Autodesk Fusion 360 part; units mm, degrees
(part 16 of 18)
  line L9589 (199.0354, -77.1606) -> (199.0354, -76.5606)
  line L9590 (199.3854, -77.1606) -> (199.0354, -77.1606)
  line L9591 (199.0354, -76.5606) -> (199.3854, -76.5606)
  line L9592 (195.5854, -58.0978) -> (195.9354, -58.0978)
  line L9593 (195.9354, -58.0978) -> (195.9354, -57.4978)
  line L9594 (195.9354, -57.4978) -> (195.5854, -57.4978)
  line L9595 (195.5854, -57.4978) -> (195.5854, -58.0978)
  line L9596 (199.0354, -57.4978) -> (199.3854, -57.4978)
  line L9597 (199.3854, -58.0978) -> (199.0354, -58.0978)
  line L9598 (199.3854, -57.4978) -> (199.3854, -58.0978)
  line L9599 (199.0354, -58.0978) -> (199.0354, -57.4978)
  line L9600 (195.5854, -19.385) -> (195.5854, -19.985)
  line L9601 (195.9354, -19.385) -> (195.5854, -19.385)
  line L9602 (195.9354, -19.985) -> (195.9354, -19.385)
  line L9603 (195.5854, -19.985) -> (195.9354, -19.985)
  line L9604 (199.3854, -19.985) -> (199.0354, -19.985)
  line L9605 (199.0354, -19.985) -> (199.0354, -19.385)
  line L9606 (199.3854, -19.385) -> (199.3854, -19.985)
  line L9607 (199.0354, -19.385) -> (199.3854, -19.385)
  line L9608 (203.2384, -3.41) -> (203.2384, -4.21)
  line L9609 (202.9384, -3.41) -> (203.2384, -3.41)
  line L9610 (202.9384, -4.21) -> (202.9384, -3.41)
  line L9611 (203.2384, -4.21) -> (202.9384, -4.21)
  line L9612 (201.9384, -4.21) -> (201.9384, -3.41)
  line L9613 (201.6384, -4.21) -> (201.9384, -4.21)
  line L9614 (201.6384, -3.41) -> (201.6384, -4.21)
  line L9615 (201.9384, -3.41) -> (201.6384, -3.41)
  line L9616 (201.0334, -7.131) -> (201.0334, -6.331)
  line L9617 (201.0334, -6.331) -> (201.3334, -6.331)
  line L9618 (201.3334, -6.331) -> (201.3334, -7.131)
  line L9619 (201.3334, -7.131) -> (201.0334, -7.131)
  line L9620 (199.7334, -7.131) -> (200.0334, -7.131)
  line L9621 (199.7334, -6.331) -> (199.7334, -7.131)
  line L9622 (200.0334, -7.131) -> (200.0334, -6.331)
  line L9623 (200.0334, -6.331) -> (199.7334, -6.331)
  line L9624 (204.9404, -4.426) -> (205.2404, -4.426)
  line L9625 (204.9404, -5.226) -> (204.9404, -4.426)
  line L9626 (205.2404, -4.426) -> (205.2404, -5.226)
  line L9627 (205.2404, -5.226) -> (204.9404, -5.226)
  line L9628 (206.5404, -5.226) -> (206.5404, -4.426)
  line L9629 (206.2404, -4.426) -> (206.2404, -5.226)
  line L9630 (206.5404, -4.426) -> (206.2404, -4.426)
  line L9631 (206.2404, -5.226) -> (206.5404, -5.226)
  line L9632 (2.9129, -0.5611) -> (1.413, -0.5611)
  line L9633 (2.9129, 0.6389) -> (2.9129, -0.5611)
  line L9634 (1.413, 0.6389) -> (2.9129, 0.6389)
  line L9635 (1.413, -0.5611) -> (1.413, 0.6389)
  line L9636 (2.9129, -10.3611) -> (2.9129, -11.5611)
  line L9637 (1.413, -11.5611) -> (1.413, -10.3611)
  line L9638 (1.413, -10.3611) -> (2.9129, -10.3611)
  line L9639 (2.9129, -11.5611) -> (1.413, -11.5611)
  line L9640 (197.1222, -3.92) -> (197.1222, -3.67)
  line L9641 (197.4822, -3.92) -> (197.1222, -3.92)
  line L9642 (197.1222, -3.67) -> (197.4822, -3.67)
  line L9643 (197.4822, -3.67) -> (197.4822, -3.92)
  line L9644 (197.4823, -4.97) -> (197.4823, -5.22)
  line L9645 (197.4823, -5.22) -> (197.1223, -5.22)
  line L9646 (197.1223, -5.22) -> (197.1223, -4.97)
  line L9647 (197.1223, -4.97) -> (197.4823, -4.97)
  line L9648 (195.5524, -3.92) -> (195.1924, -3.92)
  line L9649 (195.5524, -3.67) -> (195.5524, -3.92)
  line L9650 (195.1924, -3.67) -> (195.5524, -3.67)
  line L9651 (195.1924, -3.92) -> (195.1924, -3.67)
  line L9652 (195.1924, -4.57) -> (195.1924, -4.32)
  line L9653 (195.5524, -4.32) -> (195.5524, -4.57)
  line L9654 (195.1924, -4.32) -> (195.5524, -4.32)
  line L9655 (195.5524, -4.57) -> (195.1924, -4.57)
  line L9656 (195.5524, -4.97) -> (195.5524, -5.22)
  line L9657 (195.5524, -5.22) -> (195.1924, -5.22)
  line L9658 (195.1924, -4.97) -> (195.5524, -4.97)
  line L9659 (195.1924, -5.22) -> (195.1924, -4.97)
  line L9660 (201.1604, -2.305) -> (201.1604, -1.505)
  line L9661 (201.1604, -1.505) -> (201.4604, -1.505)
  line L9662 (201.4604, -1.505) -> (201.4604, -2.305)
  line L9663 (201.4604, -2.305) -> (201.1604, -2.305)
  line L9664 (199.8604, -2.305) -> (200.1604, -2.305)
  line L9665 (200.1604, -1.505) -> (199.8604, -1.505)
  line L9666 (200.1604, -2.305) -> (200.1604, -1.505)
  line L9667 (199.8604, -1.505) -> (199.8604, -2.305)
  line L9668 (207.5745, -6.0629) -> (207.9745, -6.0629)
  line L9669 (207.9745, -6.2629) -> (207.5745, -6.2629)
  line L9670 (207.9745, -6.0629) -> (207.9745, -6.2629)
  line L9671 (207.5745, -6.2629) -> (207.5745, -6.0629)
  line L9672 (207.9745, -6.6629) -> (207.5745, -6.6629)
  line L9673 (207.5745, -6.6629) -> (207.5745, -6.4629)
  line L9674 (207.5745, -6.4629) -> (207.9745, -6.4629)
  line L9675 (207.9745, -6.4629) -> (207.9745, -6.6629)
  line L9676 (207.5745, -6.8629) -> (207.9745, -6.8629)
  line L9677 (207.9745, -6.8629) -> (207.9745, -7.0629)
  line L9678 (207.5745, -7.0629) -> (207.5745, -6.8629)
  line L9679 (207.9745, -7.0629) -> (207.5745, -7.0629)
  line L9680 (207.5745, -7.2629) -> (207.9745, -7.2629)
  line L9681 (207.9745, -7.2629) -> (207.9745, -7.4629)
  line L9682 (207.5745, -7.4629) -> (207.5745, -7.2629)
  line L9683 (207.9745, -7.4629) -> (207.5745, -7.4629)
  line L9684 (207.5745, -7.8629) -> (207.5745, -7.6629)
  line L9685 (207.9745, -7.8629) -> (207.5745, -7.8629)
  line L9686 (207.9745, -7.6629) -> (207.9745, -7.8629)
  line L9687 (207.5745, -7.6629) -> (207.9745, -7.6629)
  line L9688 (207.9745, -8.0629) -> (207.9745, -8.2629)
  line L9689 (207.9745, -8.2629) -> (207.5745, -8.2629)
  line L9690 (207.5745, -8.2629) -> (207.5745, -8.0629)
  line L9691 (207.5745, -8.0629) -> (207.9745, -8.0629)
  line L9692 (207.9745, -8.6629) -> (207.5745, -8.6629)
  line L9693 (207.5745, -8.4629) -> (207.9745, -8.4629)
  line L9694 (207.5745, -8.6629) -> (207.5745, -8.4629)
  line L9695 (207.9745, -8.4629) -> (207.9745, -8.6629)
  line L9696 (207.5745, -8.8629) -> (207.9745, -8.8629)
  line L9697 (207.9745, -9.0629) -> (207.5745, -9.0629)
  line L9698 (207.5745, -9.0629) -> (207.5745, -8.8629)
  line L9699 (207.9745, -8.8629) -> (207.9745, -9.0629)
  line L9700 (207.5745, -9.4629) -> (207.5745, -9.2629)
  line L9701 (207.9745, -9.2629) -> (207.9745, -9.4629)
  line L9702 (207.5745, -9.2629) -> (207.9745, -9.2629)
  line L9703 (207.9745, -9.4629) -> (207.5745, -9.4629)
  line L9704 (207.5745, -9.6629) -> (207.9745, -9.6629)
  line L9705 (207.9745, -9.8629) -> (207.5745, -9.8629)
  line L9706 (207.5745, -9.8629) -> (207.5745, -9.6629)
  line L9707 (207.9745, -9.6629) -> (207.9745, -9.8629)
  line L9708 (207.5745, -10.2629) -> (207.5745, -10.0629)
  line L9709 (207.9745, -10.0629) -> (207.9745, -10.2629)
  line L9710 (207.9745, -10.2629) -> (207.5745, -10.2629)
  line L9711 (207.5745, -10.0629) -> (207.9745, -10.0629)
  line L9712 (207.9745, -10.6629) -> (207.5745, -10.6629)
  line L9713 (207.9745, -10.4629) -> (207.9745, -10.6629)
  line L9714 (207.5745, -10.6629) -> (207.5745, -10.4629)
  line L9715 (207.5745, -10.4629) -> (207.9745, -10.4629)
  line L9716 (207.5745, -10.8629) -> (207.9745, -10.8629)
  line L9717 (207.9745, -10.8629) -> (207.9745, -11.0629)
  line L9718 (207.9745, -11.0629) -> (207.5745, -11.0629)
  line L9719 (207.5745, -11.0629) -> (207.5745, -10.8629)
  line L9720 (207.9745, -11.4629) -> (207.5745, -11.4629)
  line L9721 (207.5745, -11.4629) -> (207.5745, -11.2629)
  line L9722 (207.5745, -11.2629) -> (207.9745, -11.2629)
  line L9723 (207.9745, -11.2629) -> (207.9745, -11.4629)
  line L9724 (208.5745, -12.2629) -> (208.3745, -12.2629)
  line L9725 (208.3745, -12.2629) -> (208.3745, -11.8629)
  line L9726 (208.5745, -11.8629) -> (208.5745, -12.2629)
  line L9727 (208.3745, -11.8629) -> (208.5745, -11.8629)
  line L9728 (208.9745, -12.2629) -> (208.7745, -12.2629)
  line L9729 (208.7745, -11.8629) -> (208.9745, -11.8629)
  line L9730 (208.7745, -12.2629) -> (208.7745, -11.8629)
  line L9731 (208.9745, -11.8629) -> (208.9745, -12.2629)
  line L9732 (209.3745, -11.8629) -> (209.3745, -12.2629)
  line L9733 (209.3745, -12.2629) -> (209.1745, -12.2629)
  line L9734 (209.1745, -12.2629) -> (209.1745, -11.8629)
  line L9735 (209.1745, -11.8629) -> (209.3745, -11.8629)
  line L9736 (209.5745, -11.8629) -> (209.7745, -11.8629)
  line L9737 (209.7745, -11.8629) -> (209.7745, -12.2629)
  line L9738 (209.5745, -12.2629) -> (209.5745, -11.8629)
  line L9739 (209.7745, -12.2629) -> (209.5745, -12.2629)
  line L9740 (210.1745, -11.8629) -> (210.1745, -12.2629)
  line L9741 (210.1745, -12.2629) -> (209.9745, -12.2629)
  line L9742 (209.9745, -12.2629) -> (209.9745, -11.8629)
  line L9743 (209.9745, -11.8629) -> (210.1745, -11.8629)
  line L9744 (210.3745, -11.8629) -> (210.5745, -11.8629)
  line L9745 (210.3745, -12.2629) -> (210.3745, -11.8629)
  line L9746 (210.5745, -12.2629) -> (210.3745, -12.2629)
  line L9747 (210.5745, -11.8629) -> (210.5745, -12.2629)
  line L9748 (210.7745, -11.8629) -> (210.9745, -11.8629)
  line L9749 (210.9745, -11.8629) -> (210.9745, -12.2629)
  line L9750 (210.9745, -12.2629) -> (210.7745, -12.2629)
  line L9751 (210.7745, -12.2629) -> (210.7745, -11.8629)
  line L9752 (211.1745, -11.8629) -> (211.3745, -11.8629)
  line L9753 (211.3745, -11.8629) -> (211.3745, -12.2629)
  line L9754 (211.3745, -12.2629) -> (211.1745, -12.2629)
  line L9755 (211.1745, -12.2629) -> (211.1745, -11.8629)
  line L9756 (211.7745, -11.8629) -> (211.7745, -12.2629)
  line L9757 (211.5745, -12.2629) -> (211.5745, -11.8629)
  line L9758 (211.7745, -12.2629) -> (211.5745, -12.2629)
  line L9759 (211.5745, -11.8629) -> (211.7745, -11.8629)
  line L9760 (211.9745, -12.2629) -> (211.9745, -11.8629)
  line L9761 (212.1745, -11.8629) -> (212.1745, -12.2629)
  line L9762 (212.1745, -12.2629) -> (211.9745, -12.2629)
  line L9763 (211.9745, -11.8629) -> (212.1745, -11.8629)
  line L9764 (212.3745, -12.2629) -> (212.3745, -11.8629)
  line L9765 (212.3745, -11.8629) -> (212.5745, -11.8629)
  line L9766 (212.5745, -11.8629) -> (212.5745, -12.2629)
  line L9767 (212.5745, -12.2629) -> (212.3745, -12.2629)
  line L9768 (212.7745, -12.2629) -> (212.7745, -11.8629)
  line L9769 (212.9745, -12.2629) -> (212.7745, -12.2629)
  line L9770 (212.9745, -11.8629) -> (212.9745, -12.2629)
  line L9771 (212.7745, -11.8629) -> (212.9745, -11.8629)
  line L9772 (213.3745, -12.2629) -> (213.1745, -12.2629)
  line L9773 (213.3745, -11.8629) -> (213.3745, -12.2629)
  line L9774 (213.1745, -11.8629) -> (213.3745, -11.8629)
  line L9775 (213.1745, -12.2629) -> (213.1745, -11.8629)
  line L9776 (213.7745, -12.2629) -> (213.5745, -12.2629)
  line L9777 (213.5745, -12.2629) -> (213.5745, -11.8629)
  line L9778 (213.7745, -11.8629) -> (213.7745, -12.2629)
  line L9779 (213.5745, -11.8629) -> (213.7745, -11.8629)
  line L9780 (214.5745, -11.4629) -> (214.5745, -11.2629)
  line L9781 (214.5745, -11.2629) -> (214.1745, -11.2629)
  line L9782 (214.1745, -11.2629) -> (214.1745, -11.4629)
  line L9783 (214.1745, -11.4629) -> (214.5745, -11.4629)
  line L9784 (214.5745, -11.0629) -> (214.5745, -10.8629)
  line L9785 (214.1745, -10.8629) -> (214.1745, -11.0629)
  line L9786 (214.1745, -11.0629) -> (214.5745, -11.0629)
  line L9787 (214.5745, -10.8629) -> (214.1745, -10.8629)
  line L9788 (214.5745, -10.6629) -> (214.5745, -10.4629)
  line L9789 (214.1745, -10.6629) -> (214.5745, -10.6629)
  line L9790 (214.1745, -10.4629) -> (214.1745, -10.6629)
  line L9791 (214.5745, -10.4629) -> (214.1745, -10.4629)
  line L9792 (214.5745, -10.0629) -> (214.1745, -10.0629)
  line L9793 (214.1745, -10.0629) -> (214.1745, -10.2629)
  line L9794 (214.5745, -10.2629) -> (214.5745, -10.0629)
  line L9795 (214.1745, -10.2629) -> (214.5745, -10.2629)
  line L9796 (214.1745, -9.8629) -> (214.5745, -9.8629)
  line L9797 (214.1745, -9.6629) -> (214.1745, -9.8629)
  line L9798 (214.5745, -9.8629) -> (214.5745, -9.6629)
  line L9799 (214.5745, -9.6629) -> (214.1745, -9.6629)
  line L9800 (214.1745, -9.4629) -> (214.5745, -9.4629)
  line L9801 (214.5745, -9.4629) -> (214.5745, -9.2629)
  line L9802 (214.1745, -9.2629) -> (214.1745, -9.4629)
  line L9803 (214.5745, -9.2629) -> (214.1745, -9.2629)
  line L9804 (214.1745, -8.8629) -> (214.1745, -9.0629)
  line L9805 (214.5745, -8.8629) -> (214.1745, -8.8629)
  line L9806 (214.1745, -9.0629) -> (214.5745, -9.0629)
  line L9807 (214.5745, -9.0629) -> (214.5745, -8.8629)
  line L9808 (214.1745, -8.6629) -> (214.5745, -8.6629)
  line L9809 (214.5745, -8.4629) -> (214.1745, -8.4629)
  line L9810 (214.5745, -8.6629) -> (214.5745, -8.4629)
  line L9811 (214.1745, -8.4629) -> (214.1745, -8.6629)
  line L9812 (214.1745, -8.2629) -> (214.5745, -8.2629)
  line L9813 (214.5745, -8.0629) -> (214.1745, -8.0629)
  line L9814 (214.1745, -8.0629) -> (214.1745, -8.2629)
  line L9815 (214.5745, -8.2629) -> (214.5745, -8.0629)
  line L9816 (214.5745, -7.6629) -> (214.1745, -7.6629)
  line L9817 (214.1745, -7.6629) -> (214.1745, -7.8629)
  line L9818 (214.1745, -7.8629) -> (214.5745, -7.8629)
  line L9819 (214.5745, -7.8629) -> (214.5745, -7.6629)
  line L9820 (214.5745, -7.2629) -> (214.1745, -7.2629)
  line L9821 (214.1745, -7.2629) -> (214.1745, -7.4629)
  line L9822 (214.5745, -7.4629) -> (214.5745, -7.2629)
  line L9823 (214.1745, -7.4629) -> (214.5745, -7.4629)
  line L9824 (214.1745, -7.0629) -> (214.5745, -7.0629)
  line L9825 (214.1745, -6.8629) -> (214.1745, -7.0629)
  line L9826 (214.5745, -7.0629) -> (214.5745, -6.8629)
  line L9827 (214.5745, -6.8629) -> (214.1745, -6.8629)
  line L9828 (214.5745, -6.4629) -> (214.1745, -6.4629)
  line L9829 (214.1745, -6.4629) -> (214.1745, -6.6629)
  line L9830 (214.5745, -6.6629) -> (214.5745, -6.4629)
  line L9831 (214.1745, -6.6629) -> (214.5745, -6.6629)
  line L9832 (214.1745, -6.2629) -> (214.5745, -6.2629)
  line L9833 (214.5745, -6.0629) -> (214.1745, -6.0629)
  line L9834 (214.5745, -6.2629) -> (214.5745, -6.0629)
  line L9835 (214.1745, -6.0629) -> (214.1745, -6.2629)
  line L9836 (213.7745, -5.2629) -> (213.5745, -5.2629)
  line L9837 (213.7745, -5.6629) -> (213.7745, -5.2629)
  line L9838 (213.5745, -5.2629) -> (213.5745, -5.6629)
  line L9839 (213.5745, -5.6629) -> (213.7745, -5.6629)
  line L9840 (213.1745, -5.6629) -> (213.3745, -5.6629)
  line L9841 (213.1745, -5.2629) -> (213.1745, -5.6629)
  line L9842 (213.3745, -5.2629) -> (213.1745, -5.2629)
  line L9843 (213.3745, -5.6629) -> (213.3745, -5.2629)
  line L9844 (212.7745, -5.6629) -> (212.9745, -5.6629)
  line L9845 (212.7745, -5.2629) -> (212.7745, -5.6629)
  line L9846 (212.9745, -5.2629) -> (212.7745, -5.2629)
  line L9847 (212.9745, -5.6629) -> (212.9745, -5.2629)
  line L9848 (212.3745, -5.6629) -> (212.5745, -5.6629)
  line L9849 (212.5745, -5.6629) -> (212.5745, -5.2629)
  line L9850 (212.3745, -5.2629) -> (212.3745, -5.6629)
  line L9851 (212.5745, -5.2629) -> (212.3745, -5.2629)
  line L9852 (212.1745, -5.6629) -> (212.1745, -5.2629)
  line L9853 (211.9745, -5.6629) -> (212.1745, -5.6629)
  line L9854 (211.9745, -5.2629) -> (211.9745, -5.6629)
  line L9855 (212.1745, -5.2629) -> (211.9745, -5.2629)
  line L9856 (211.5745, -5.2629) -> (211.5745, -5.6629)
  line L9857 (211.7745, -5.6629) -> (211.7745, -5.2629)
  line L9858 (211.5745, -5.6629) -> (211.7745, -5.6629)
  line L9859 (211.7745, -5.2629) -> (211.5745, -5.2629)
  line L9860 (211.1745, -5.6629) -> (211.3745, -5.6629)
  line L9861 (211.3745, -5.2629) -> (211.1745, -5.2629)
  line L9862 (211.1745, -5.2629) -> (211.1745, -5.6629)
  line L9863 (211.3745, -5.6629) -> (211.3745, -5.2629)
  line L9864 (210.9745, -5.2629) -> (210.7745, -5.2629)
  line L9865 (210.7745, -5.6629) -> (210.9745, -5.6629)
  line L9866 (210.9745, -5.6629) -> (210.9745, -5.2629)
  line L9867 (210.7745, -5.2629) -> (210.7745, -5.6629)
  line L9868 (210.3745, -5.2629) -> (210.3745, -5.6629)
  line L9869 (210.3745, -5.6629) -> (210.5745, -5.6629)
  line L9870 (210.5745, -5.2629) -> (210.3745, -5.2629)
  line L9871 (210.5745, -5.6629) -> (210.5745, -5.2629)
  line L9872 (209.9745, -5.2629) -> (209.9745, -5.6629)
  line L9873 (209.9745, -5.6629) -> (210.1745, -5.6629)
  line L9874 (210.1745, -5.6629) -> (210.1745, -5.2629)
  line L9875 (210.1745, -5.2629) -> (209.9745, -5.2629)
  line L9876 (209.5745, -5.6629) -> (209.7745, -5.6629)
  line L9877 (209.5745, -5.2629) -> (209.5745, -5.6629)
  line L9878 (209.7745, -5.2629) -> (209.5745, -5.2629)
  line L9879 (209.7745, -5.6629) -> (209.7745, -5.2629)
  line L9880 (209.1745, -5.2629) -> (209.1745, -5.6629)
  line L9881 (209.1745, -5.6629) -> (209.3745, -5.6629)
  line L9882 (209.3745, -5.6629) -> (209.3745, -5.2629)
  line L9883 (209.3745, -5.2629) -> (209.1745, -5.2629)
  line L9884 (208.9745, -5.2629) -> (208.7745, -5.2629)
  line L9885 (208.7745, -5.6629) -> (208.9745, -5.6629)
  line L9886 (208.9745, -5.6629) -> (208.9745, -5.2629)
  line L9887 (208.7745, -5.2629) -> (208.7745, -5.6629)
  line L9888 (208.3745, -5.2629) -> (208.3745, -5.6629)
  line L9889 (208.3745, -5.6629) -> (208.5745, -5.6629)
  line L9890 (208.5745, -5.2629) -> (208.3745, -5.2629)
  line L9891 (208.5745, -5.6629) -> (208.5745, -5.2629)
  line L9892 (209.0745, -6.7629) -> (213.0745, -6.7629)
  line L9893 (209.0745, -10.7629) -> (209.0745, -6.7629)
  line L9894 (213.0745, -6.7629) -> (213.0745, -10.7629)
  line L9895 (213.0745, -10.7629) -> (209.0745, -10.7629)
  line L9896 (187.2064, -6.331) -> (187.2064, -7.131)
  line L9897 (186.9064, -7.131) -> (186.9064, -6.331)
  line L9898 (187.2064, -7.131) -> (186.9064, -7.131)
  line L9899 (186.9064, -6.331) -> (187.2064, -6.331)
  line L9900 (188.2064, -6.331) -> (188.2064, -7.131)
  line L9901 (188.5064, -6.331) -> (188.2064, -6.331)
  line L9902 (188.2064, -7.131) -> (188.5064, -7.131)
  line L9903 (188.5064, -7.131) -> (188.5064, -6.331)
  line L9904 (183.6344, -6.331) -> (183.9344, -6.331)
  line L9905 (183.9344, -6.331) -> (183.9344, -7.131)
  line L9906 (183.6344, -7.131) -> (183.6344, -6.331)
  line L9907 (183.9344, -7.131) -> (183.6344, -7.131)
  line L9908 (182.3344, -7.131) -> (182.6344, -7.131)
  line L9909 (182.3344, -6.331) -> (182.3344, -7.131)
  line L9910 (182.6344, -6.331) -> (182.3344, -6.331)
  line L9911 (182.6344, -7.131) -> (182.6344, -6.331)
  line L9912 (207.7354, -3.1661) -> (208.2854, -3.1661)
  line L9913 (207.7354, -3.4061) -> (207.7354, -3.1661)
  line L9914 (208.2854, -3.1661) -> (208.2854, -3.4061)
  line L9915 (208.2854, -3.4061) -> (207.7354, -3.4061)
  line L9916 (208.2854, -2.906) -> (207.7354, -2.906)
  line L9917 (207.7354, -2.666) -> (208.2854, -2.666)
  line L9918 (207.7354, -2.906) -> (207.7354, -2.666)
  line L9919 (208.2854, -2.666) -> (208.2854, -2.906)
  line L9920 (208.2854, -2.1659) -> (208.2854, -2.4059)
  line L9921 (208.2854, -2.4059) -> (207.7354, -2.4059)
  line L9922 (207.7354, -2.4059) -> (207.7354, -2.1659)
  line L9923 (207.7354, -2.1659) -> (208.2854, -2.1659)
  line L9924 (208.2854, -1.906) -> (207.7354, -1.906)
  line L9925 (207.7354, -1.666) -> (208.2854, -1.666)
  line L9926 (208.2854, -1.666) -> (208.2854, -1.906)
  line L9927 (207.7354, -1.906) -> (207.7354, -1.666)
  line L9928 (208.2854, -1.1661) -> (208.2854, -1.4061)
  line L9929 (207.7354, -1.1661) -> (208.2854, -1.1661)
  line L9930 (208.2854, -1.4061) -> (207.7354, -1.4061)
  line L9931 (207.7354, -1.4061) -> (207.7354, -1.1661)
  line L9932 (212.6354, -1.4059) -> (212.0854, -1.4059)
  line L9933 (212.0854, -1.4059) -> (212.0854, -1.1659)
  line L9934 (212.6354, -1.1659) -> (212.6354, -1.4059)
  line L9935 (212.0854, -1.1659) -> (212.6354, -1.1659)
  line L9936 (212.6354, -1.906) -> (212.0854, -1.906)
  line L9937 (212.6354, -1.666) -> (212.6354, -1.906)
  line L9938 (212.0854, -1.666) -> (212.6354, -1.666)
  line L9939 (212.0854, -1.906) -> (212.0854, -1.666)
  line L9940 (212.0854, -2.4061) -> (212.0854, -2.1661)
  line L9941 (212.0854, -2.1661) -> (212.6354, -2.1661)
  line L9942 (212.6354, -2.1661) -> (212.6354, -2.4061)
  line L9943 (212.6354, -2.4061) -> (212.0854, -2.4061)
  line L9944 (212.0854, -2.666) -> (212.6354, -2.666)
  line L9945 (212.6354, -2.906) -> (212.0854, -2.906)
  line L9946 (212.6354, -2.666) -> (212.6354, -2.906)
  line L9947 (212.0854, -2.906) -> (212.0854, -2.666)
  line L9948 (212.0854, -3.4059) -> (212.0854, -3.1659)
  line L9949 (212.0854, -3.1659) -> (212.6354, -3.1659)
  line L9950 (212.6354, -3.4059) -> (212.0854, -3.4059)
  line L9951 (212.6354, -3.1659) -> (212.6354, -3.4059)
  line L9952 (138.4353, -76.5606) -> (138.4353, -77.1606)
  line L9953 (138.7853, -76.5606) -> (138.4353, -76.5606)
  line L9954 (138.4353, -77.1606) -> (138.7853, -77.1606)
  line L9955 (138.7853, -77.1606) -> (138.7853, -76.5606)
  line L9956 (141.8853, -77.1606) -> (141.8853, -76.5606)
  line L9957 (141.8853, -76.5606) -> (142.2353, -76.5606)
  line L9958 (142.2353, -77.1606) -> (141.8853, -77.1606)
  line L9959 (142.2353, -76.5606) -> (142.2353, -77.1606)
  line L9960 (138.4353, -19.385) -> (138.4353, -19.985)
  line L9961 (138.7853, -19.385) -> (138.4353, -19.385)
  line L9962 (138.7853, -19.985) -> (138.7853, -19.385)
  line L9963 (138.4353, -19.985) -> (138.7853, -19.985)
  line L9964 (141.8853, -19.385) -> (142.2353, -19.385)
  line L9965 (142.2353, -19.385) -> (142.2353, -19.985)
  line L9966 (142.2353, -19.985) -> (141.8853, -19.985)
  line L9967 (141.8853, -19.985) -> (141.8853, -19.385)
  line L9968 (138.7853, -39.0351) -> (138.7853, -38.4351)
  line L9969 (138.7853, -38.4351) -> (138.4353, -38.4351)
  line L9970 (138.4353, -38.4351) -> (138.4353, -39.0351)
  line L9971 (138.4353, -39.0351) -> (138.7853, -39.0351)
  line L9972 (141.8853, -38.4351) -> (142.2353, -38.4351)
  line L9973 (142.2353, -38.4351) -> (142.2353, -39.0351)
  line L9974 (141.8853, -39.0351) -> (141.8853, -38.4351)
  line L9975 (142.2353, -39.0351) -> (141.8853, -39.0351)
  line L9976 (138.4353, -58.0978) -> (138.7853, -58.0978)
  line L9977 (138.7853, -57.4978) -> (138.4353, -57.4978)
  line L9978 (138.7853, -58.0978) -> (138.7853, -57.4978)
  line L9979 (138.4353, -57.4978) -> (138.4353, -58.0978)
  line L9980 (142.2353, -58.0978) -> (141.8853, -58.0978)
  line L9981 (141.8853, -57.4978) -> (142.2353, -57.4978)
  line L9982 (141.8853, -58.0978) -> (141.8853, -57.4978)
  line L9983 (142.2353, -57.4978) -> (142.2353, -58.0978)
  line L9984 (157.8353, -19.985) -> (157.8353, -19.385)
  line L9985 (157.4853, -19.985) -> (157.8353, -19.985)
  line L9986 (157.4853, -19.385) -> (157.4853, -19.985)
  line L9987 (157.8353, -19.385) -> (157.4853, -19.385)
  line L9988 (160.9353, -19.985) -> (160.9353, -19.385)
  line L9989 (161.2853, -19.985) -> (160.9353, -19.985)
  line L9990 (161.2853, -19.385) -> (161.2853, -19.985)
  line L9991 (160.9353, -19.385) -> (161.2853, -19.385)
  line L9992 (157.4853, -76.5606) -> (157.4853, -77.1606)
  line L9993 (157.8353, -77.1606) -> (157.8353, -76.5606)
  line L9994 (157.4853, -77.1606) -> (157.8353, -77.1606)
  line L9995 (157.8353, -76.5606) -> (157.4853, -76.5606)
  line L9996 (160.9353, -76.5606) -> (161.2853, -76.5606)
  line L9997 (161.2853, -76.5606) -> (161.2853, -77.1606)
  line L9998 (161.2853, -77.1606) -> (160.9353, -77.1606)
  line L9999 (160.9353, -77.1606) -> (160.9353, -76.5606)
  line L10000 (157.4853, -58.0978) -> (157.8353, -58.0978)
  line L10001 (157.8353, -58.0978) -> (157.8353, -57.4978)
  line L10002 (157.4853, -57.4978) -> (157.4853, -58.0978)
  line L10003 (157.8353, -57.4978) -> (157.4853, -57.4978)
  line L10004 (160.9353, -58.0978) -> (160.9353, -57.4978)
  line L10005 (160.9353, -57.4978) -> (161.2853, -57.4978)
  line L10006 (161.2853, -58.0978) -> (160.9353, -58.0978)
  line L10007 (161.2853, -57.4978) -> (161.2853, -58.0978)
  line L10008 (157.8353, -38.4351) -> (157.4853, -38.4351)
  line L10009 (157.4853, -39.0351) -> (157.8353, -39.0351)
  line L10010 (157.4853, -38.4351) -> (157.4853, -39.0351)
  line L10011 (157.8353, -39.0351) -> (157.8353, -38.4351)
  line L10012 (161.2853, -38.4351) -> (161.2853, -39.0351)
  line L10013 (160.9353, -38.4351) -> (161.2853, -38.4351)
  line L10014 (160.9353, -39.0351) -> (160.9353, -38.4351)
  line L10015 (161.2853, -39.0351) -> (160.9353, -39.0351)
  line L10016 (176.5354, -19.385) -> (176.5354, -19.985)
  line L10017 (176.8854, -19.985) -> (176.8854, -19.385)
  line L10018 (176.8854, -19.385) -> (176.5354, -19.385)
  line L10019 (176.5354, -19.985) -> (176.8854, -19.985)
  line L10020 (180.3354, -19.985) -> (179.9854, -19.985)
  line L10021 (180.3354, -19.385) -> (180.3354, -19.985)
  line L10022 (179.9854, -19.985) -> (179.9854, -19.385)
  line L10023 (179.9854, -19.385) -> (180.3354, -19.385)
  line L10024 (176.8854, -76.5606) -> (176.5354, -76.5606)
  line L10025 (176.8854, -77.1606) -> (176.8854, -76.5606)
  line L10026 (176.5354, -76.5606) -> (176.5354, -77.1606)
  line L10027 (176.5354, -77.1606) -> (176.8854, -77.1606)
  line L10028 (180.3354, -76.5606) -> (180.3354, -77.1606)
  line L10029 (179.9854, -76.5606) -> (180.3354, -76.5606)
  line L10030 (179.9854, -77.1606) -> (179.9854, -76.5606)
  line L10031 (180.3354, -77.1606) -> (179.9854, -77.1606)
  line L10032 (176.8854, -58.0978) -> (176.8854, -57.4978)
  line L10033 (176.5354, -58.0978) -> (176.8854, -58.0978)
  line L10034 (176.5354, -57.4978) -> (176.5354, -58.0978)
  line L10035 (176.8854, -57.4978) -> (176.5354, -57.4978)
  line L10036 (179.9854, -58.0978) -> (179.9854, -57.4978)
  line L10037 (180.3354, -58.0978) -> (179.9854, -58.0978)
  line L10038 (179.9854, -57.4978) -> (180.3354, -57.4978)
  line L10039 (180.3354, -57.4978) -> (180.3354, -58.0978)
  line L10040 (176.8854, -39.0351) -> (176.8854, -38.4351)
  line L10041 (176.5354, -38.4351) -> (176.5354, -39.0351)
  line L10042 (176.5354, -39.0351) -> (176.8854, -39.0351)
  line L10043 (176.8854, -38.4351) -> (176.5354, -38.4351)
  line L10044 (179.9854, -38.4351) -> (180.3354, -38.4351)
  line L10045 (180.3354, -39.0351) -> (179.9854, -39.0351)
  line L10046 (180.3354, -38.4351) -> (180.3354, -39.0351)
  line L10047 (179.9854, -39.0351) -> (179.9854, -38.4351)
  line L10048 (100.3352, -77.1606) -> (100.6852, -77.1606)
  line L10049 (100.3352, -76.5606) -> (100.3352, -77.1606)
  line L10050 (100.6852, -77.1606) -> (100.6852, -76.5606)
  line L10051 (100.6852, -76.5606) -> (100.3352, -76.5606)
  line L10052 (103.7852, -77.1606) -> (103.7852, -76.5606)
  line L10053 (103.7852, -76.5606) -> (104.1352, -76.5606)
  line L10054 (104.1352, -76.5606) -> (104.1352, -77.1606)
  line L10055 (104.1352, -77.1606) -> (103.7852, -77.1606)
  line L10056 (100.6852, -57.4978) -> (100.3352, -57.4978)
  line L10057 (100.3352, -57.4978) -> (100.3352, -58.0978)
  line L10058 (100.3352, -58.0978) -> (100.6852, -58.0978)
  line L10059 (100.6852, -58.0978) -> (100.6852, -57.4978)
  line L10060 (103.7852, -57.4978) -> (104.1352, -57.4978)
  line L10061 (104.1352, -58.0978) -> (103.7852, -58.0978)
  line L10062 (103.7852, -58.0978) -> (103.7852, -57.4978)
  line L10063 (104.1352, -57.4978) -> (104.1352, -58.0978)
  line L10064 (100.6852, -19.385) -> (100.3352, -19.385)
  line L10065 (100.6852, -19.985) -> (100.6852, -19.385)
  line L10066 (100.3352, -19.985) -> (100.6852, -19.985)
  line L10067 (100.3352, -19.385) -> (100.3352, -19.985)
  line L10068 (104.1352, -19.985) -> (103.7852, -19.985)
  line L10069 (104.1352, -19.385) -> (104.1352, -19.985)
  line L10070 (103.7852, -19.385) -> (104.1352, -19.385)
  line L10071 (103.7852, -19.985) -> (103.7852, -19.385)
  line L10072 (100.3352, -38.4351) -> (100.3352, -39.0351)
  line L10073 (100.6852, -38.4351) -> (100.3352, -38.4351)
  line L10074 (100.6852, -39.0351) -> (100.6852, -38.4351)
  line L10075 (100.3352, -39.0351) -> (100.6852, -39.0351)
  line L10076 (103.7852, -38.4351) -> (104.1352, -38.4351)
  line L10077 (104.1352, -39.0351) -> (103.7852, -39.0351)
  line L10078 (104.1352, -38.4351) -> (104.1352, -39.0351)
  line L10079 (103.7852, -39.0351) -> (103.7852, -38.4351)
  line L10080 (119.3852, -19.385) -> (119.3852, -19.985)
  line L10081 (119.3852, -19.985) -> (119.7352, -19.985)
  line L10082 (119.7352, -19.385) -> (119.3852, -19.385)
  line L10083 (119.7352, -19.985) -> (119.7352, -19.385)
  line L10084 (123.1852, -19.385) -> (123.1852, -19.985)
  line L10085 (122.8352, -19.985) -> (122.8352, -19.385)
  line L10086 (122.8352, -19.385) -> (123.1852, -19.385)
  line L10087 (123.1852, -19.985) -> (122.8352, -19.985)
  line L10088 (119.3852, -58.0978) -> (119.7352, -58.0978)
  line L10089 (119.3852, -57.4978) -> (119.3852, -58.0978)
  line L10090 (119.7352, -58.0978) -> (119.7352, -57.4978)
  line L10091 (119.7352, -57.4978) -> (119.3852, -57.4978)
  line L10092 (123.1852, -57.4978) -> (123.1852, -58.0978)
  line L10093 (122.8352, -58.0978) -> (122.8352, -57.4978)
  line L10094 (123.1852, -58.0978) -> (122.8352, -58.0978)
  line L10095 (122.8352, -57.4978) -> (123.1852, -57.4978)
  line L10096 (119.7352, -39.0351) -> (119.7352, -38.4351)
  line L10097 (119.3852, -38.4351) -> (119.3852, -39.0351)
  line L10098 (119.7352, -38.4351) -> (119.3852, -38.4351)
  line L10099 (119.3852, -39.0351) -> (119.7352, -39.0351)
  line L10100 (123.1852, -39.0351) -> (122.8352, -39.0351)
  line L10101 (123.1852, -38.4351) -> (123.1852, -39.0351)
  line L10102 (122.8352, -38.4351) -> (123.1852, -38.4351)
  line L10103 (122.8352, -39.0351) -> (122.8352, -38.4351)
  line L10104 (119.7352, -77.1606) -> (119.7352, -76.5606)
  line L10105 (119.3852, -76.5606) -> (119.3852, -77.1606)
  line L10106 (119.7352, -76.5606) -> (119.3852, -76.5606)
  line L10107 (119.3852, -77.1606) -> (119.7352, -77.1606)
  line L10108 (122.8352, -76.5606) -> (123.1852, -76.5606)
  line L10109 (123.1852, -77.1606) -> (122.8352, -77.1606)
  line L10110 (122.8352, -77.1606) -> (122.8352, -76.5606)
  line L10111 (123.1852, -76.5606) -> (123.1852, -77.1606)
  line L10112 (5.085, -76.5606) -> (5.085, -77.1606)
  line L10113 (5.085, -77.1606) -> (5.435, -77.1606)
  line L10114 (5.435, -76.5606) -> (5.085, -76.5606)
  line L10115 (5.435, -77.1606) -> (5.435, -76.5606)
  line L10116 (8.885, -77.1606) -> (8.535, -77.1606)
  line L10117 (8.535, -76.5606) -> (8.885, -76.5606)
  line L10118 (8.535, -77.1606) -> (8.535, -76.5606)
  line L10119 (8.885, -76.5606) -> (8.885, -77.1606)
  line L10120 (24.4851, -76.5606) -> (24.1351, -76.5606)
  line L10121 (24.4851, -77.1606) -> (24.4851, -76.5606)
  line L10122 (24.1351, -76.5606) -> (24.1351, -77.1606)
  line L10123 (24.1351, -77.1606) -> (24.4851, -77.1606)
  line L10124 (27.5851, -77.1606) -> (27.5851, -76.5606)
  line L10125 (27.9351, -76.5606) -> (27.9351, -77.1606)
  line L10126 (27.5851, -76.5606) -> (27.9351, -76.5606)
  line L10127 (27.9351, -77.1606) -> (27.5851, -77.1606)
  line L10128 (43.1851, -77.1606) -> (43.5351, -77.1606)
  line L10129 (43.1851, -76.5606) -> (43.1851, -77.1606)
  line L10130 (43.5351, -76.5606) -> (43.1851, -76.5606)
  line L10131 (43.5351, -77.1606) -> (43.5351, -76.5606)
  line L10132 (46.6351, -76.5606) -> (46.9851, -76.5606)
  line L10133 (46.6351, -77.1606) -> (46.6351, -76.5606)
  line L10134 (46.9851, -77.1606) -> (46.6351, -77.1606)
  line L10135 (46.9851, -76.5606) -> (46.9851, -77.1606)
  line L10136 (62.2351, -19.385) -> (62.2351, -19.985)
  line L10137 (62.2351, -19.985) -> (62.5851, -19.985)
  line L10138 (62.5851, -19.985) -> (62.5851, -19.385)
  line L10139 (62.5851, -19.385) -> (62.2351, -19.385)
  line L10140 (66.0351, -19.985) -> (65.6851, -19.985)
  line L10141 (65.6851, -19.385) -> (66.0351, -19.385)
  line L10142 (65.6851, -19.985) -> (65.6851, -19.385)
  line L10143 (66.0351, -19.385) -> (66.0351, -19.985)
  line L10144 (62.2351, -77.1606) -> (62.5851, -77.1606)
  line L10145 (62.5851, -77.1606) -> (62.5851, -76.5606)
  line L10146 (62.5851, -76.5606) -> (62.2351, -76.5606)
  line L10147 (62.2351, -76.5606) -> (62.2351, -77.1606)
  line L10148 (65.6851, -76.5606) -> (66.0351, -76.5606)
  line L10149 (65.6851, -77.1606) -> (65.6851, -76.5606)
  line L10150 (66.0351, -77.1606) -> (65.6851, -77.1606)
  line L10151 (66.0351, -76.5606) -> (66.0351, -77.1606)
  line L10152 (62.2351, -38.4351) -> (62.2351, -39.0351)
  line L10153 (62.5851, -38.4351) -> (62.2351, -38.4351)
  line L10154 (62.5851, -39.0351) -> (62.5851, -38.4351)
  line L10155 (62.2351, -39.0351) -> (62.5851, -39.0351)
  line L10156 (65.6851, -38.4351) -> (66.0351, -38.4351)
  line L10157 (66.0351, -38.4351) -> (66.0351, -39.0351)
  line L10158 (65.6851, -39.0351) -> (65.6851, -38.4351)
  line L10159 (66.0351, -39.0351) -> (65.6851, -39.0351)
  line L10160 (62.2351, -57.4978) -> (62.2351, -58.0978)
  line L10161 (62.2351, -58.0978) -> (62.5851, -58.0978)
  line L10162 (62.5851, -57.4978) -> (62.2351, -57.4978)
  line L10163 (62.5851, -58.0978) -> (62.5851, -57.4978)
  line L10164 (66.0351, -57.4978) -> (66.0351, -58.0978)
  line L10165 (65.6851, -57.4978) -> (66.0351, -57.4978)
  line L10166 (66.0351, -58.0978) -> (65.6851, -58.0978)
  line L10167 (65.6851, -58.0978) -> (65.6851, -57.4978)
  line L10168 (81.6352, -39.0351) -> (81.6352, -38.4351)
  line L10169 (81.6352, -38.4351) -> (81.2852, -38.4351)
  line L10170 (81.2852, -39.0351) -> (81.6352, -39.0351)
  line L10171 (81.2852, -38.4351) -> (81.2852, -39.0351)
  line L10172 (85.0852, -38.4351) -> (85.0852, -39.0351)
  line L10173 (84.7352, -39.0351) -> (84.7352, -38.4351)
  line L10174 (84.7352, -38.4351) -> (85.0852, -38.4351)
  line L10175 (85.0852, -39.0351) -> (84.7352, -39.0351)
  line L10176 (81.2852, -77.1606) -> (81.6352, -77.1606)
  line L10177 (81.6352, -77.1606) -> (81.6352, -76.5606)
  line L10178 (81.6352, -76.5606) -> (81.2852, -76.5606)
  line L10179 (81.2852, -76.5606) -> (81.2852, -77.1606)
  line L10180 (85.0852, -76.5606) -> (85.0852, -77.1606)
  line L10181 (85.0852, -77.1606) -> (84.7352, -77.1606)
  line L10182 (84.7352, -76.5606) -> (85.0852, -76.5606)
  line L10183 (84.7352, -77.1606) -> (84.7352, -76.5606)
  line L10184 (81.6352, -19.985) -> (81.6352, -19.385)
  line L10185 (81.6352, -19.385) -> (81.2852, -19.385)
  line L10186 (81.2852, -19.985) -> (81.6352, -19.985)
  line L10187 (81.2852, -19.385) -> (81.2852, -19.985)
  line L10188 (84.7352, -19.385) -> (85.0852, -19.385)
  line L10189 (84.7352, -19.985) -> (84.7352, -19.385)
  line L10190 (85.0852, -19.985) -> (84.7352, -19.985)
  line L10191 (85.0852, -19.385) -> (85.0852, -19.985)
  line L10192 (81.2852, -58.0978) -> (81.6352, -58.0978)
  line L10193 (81.2852, -57.4978) -> (81.2852, -58.0978)
  line L10194 (81.6352, -58.0978) -> (81.6352, -57.4978)
  line L10195 (81.6352, -57.4978) -> (81.2852, -57.4978)
  line L10196 (85.0852, -58.0978) -> (84.7352, -58.0978)
  line L10197 (84.7352, -58.0978) -> (84.7352, -57.4978)
  line L10198 (84.7352, -57.4978) -> (85.0852, -57.4978)
  line L10199 (85.0852, -57.4978) -> (85.0852, -58.0978)
  line L10200 (5.085, -57.4978) -> (5.085, -58.0978)
  line L10201 (5.085, -58.0978) -> (5.435, -58.0978)
  line L10202 (5.435, -57.4978) -> (5.085, -57.4978)
  line L10203 (5.435, -58.0978) -> (5.435, -57.4978)
  line L10204 (8.885, -57.4978) -> (8.885, -58.0978)
  line L10205 (8.885, -58.0978) -> (8.535, -58.0978)
  line L10206 (8.535, -57.4978) -> (8.885, -57.4978)
  line L10207 (8.535, -58.0978) -> (8.535, -57.4978)
  line L10208 (5.085, -19.985) -> (5.435, -19.985)
  line L10209 (5.435, -19.385) -> (5.085, -19.385)
  line L10210 (5.435, -19.985) -> (5.435, -19.385)
  line L10211 (5.085, -19.385) -> (5.085, -19.985)
  line L10212 (8.885, -19.985) -> (8.535, -19.985)
  line L10213 (8.535, -19.985) -> (8.535, -19.385)
  line L10214 (8.535, -19.385) -> (8.885, -19.385)
  line L10215 (8.885, -19.385) -> (8.885, -19.985)
  line L10216 (5.435, -39.0351) -> (5.435, -38.4351)
  line L10217 (5.085, -38.4351) -> (5.085, -39.0351)
  line L10218 (5.085, -39.0351) -> (5.435, -39.0351)
  line L10219 (5.435, -38.4351) -> (5.085, -38.4351)
  line L10220 (8.535, -38.4351) -> (8.885, -38.4351)
  line L10221 (8.535, -39.0351) -> (8.535, -38.4351)
  line L10222 (8.885, -39.0351) -> (8.535, -39.0351)
  line L10223 (8.885, -38.4351) -> (8.885, -39.0351)
  line L10224 (24.4851, -39.0351) -> (24.4851, -38.4351)
  line L10225 (24.4851, -38.4351) -> (24.1351, -38.4351)
  line L10226 (24.1351, -39.0351) -> (24.4851, -39.0351)
  line L10227 (24.1351, -38.4351) -> (24.1351, -39.0351)
  line L10228 (27.9351, -38.4351) -> (27.9351, -39.0351)
  line L10229 (27.9351, -39.0351) -> (27.5851, -39.0351)
  line L10230 (27.5851, -39.0351) -> (27.5851, -38.4351)
  line L10231 (27.5851, -38.4351) -> (27.9351, -38.4351)
  line L10232 (24.4851, -19.985) -> (24.4851, -19.385)
  line L10233 (24.1351, -19.385) -> (24.1351, -19.985)
  line L10234 (24.1351, -19.985) -> (24.4851, -19.985)
  line L10235 (24.4851, -19.385) -> (24.1351, -19.385)
  line L10236 (27.5851, -19.385) -> (27.9351, -19.385)
  line L10237 (27.9351, -19.385) -> (27.9351, -19.985)
  line L10238 (27.9351, -19.985) -> (27.5851, -19.985)
  line L10239 (27.5851, -19.985) -> (27.5851, -19.385)
  line L10240 (24.4851, -57.4978) -> (24.1351, -57.4978)
  line L10241 (24.4851, -58.0978) -> (24.4851, -57.4978)
  line L10242 (24.1351, -57.4978) -> (24.1351, -58.0978)
  line L10243 (24.1351, -58.0978) -> (24.4851, -58.0978)
  line L10244 (27.9351, -58.0978) -> (27.5851, -58.0978)
  line L10245 (27.9351, -57.4978) -> (27.9351, -58.0978)
  line L10246 (27.5851, -58.0978) -> (27.5851, -57.4978)
  line L10247 (27.5851, -57.4978) -> (27.9351, -57.4978)
  line L10248 (43.5351, -19.385) -> (43.1851, -19.385)
  line L10249 (43.5351, -19.985) -> (43.5351, -19.385)
  line L10250 (43.1851, -19.385) -> (43.1851, -19.985)
  line L10251 (43.1851, -19.985) -> (43.5351, -19.985)
  line L10252 (46.9851, -19.985) -> (46.6351, -19.985)
  line L10253 (46.9851, -19.385) -> (46.9851, -19.985)
  line L10254 (46.6351, -19.385) -> (46.9851, -19.385)
  line L10255 (46.6351, -19.985) -> (46.6351, -19.385)
  line L10256 (43.5351, -57.4978) -> (43.1851, -57.4978)
  line L10257 (43.1851, -58.0978) -> (43.5351, -58.0978)
  line L10258 (43.1851, -57.4978) -> (43.1851, -58.0978)
  line L10259 (43.5351, -58.0978) -> (43.5351, -57.4978)
  line L10260 (46.6351, -57.4978) -> (46.9851, -57.4978)
  line L10261 (46.6351, -58.0978) -> (46.6351, -57.4978)
  line L10262 (46.9851, -57.4978) -> (46.9851, -58.0978)
  line L10263 (46.9851, -58.0978) -> (46.6351, -58.0978)
  line L10264 (43.1851, -38.4351) -> (43.1851, -39.0351)
  line L10265 (43.5351, -38.4351) -> (43.1851, -38.4351)
  line L10266 (43.1851, -39.0351) -> (43.5351, -39.0351)
  line L10267 (43.5351, -39.0351) -> (43.5351, -38.4351)
  line L10268 (46.9851, -39.0351) -> (46.6351, -39.0351)
  line L10269 (46.6351, -39.0351) -> (46.6351, -38.4351)
  line L10270 (46.9851, -38.4351) -> (46.9851, -39.0351)
  line L10271 (46.6351, -38.4351) -> (46.9851, -38.4351)
  line L10272 (214.9854, -19.985) -> (214.9854, -19.385)
  line L10273 (214.6354, -19.385) -> (214.6354, -19.985)
  line L10274 (214.6354, -19.985) -> (214.9854, -19.985)
  line L10275 (214.9854, -19.385) -> (214.6354, -19.385)
  line L10276 (218.4354, -19.985) -> (218.0854, -19.985)
  line L10277 (218.0854, -19.385) -> (218.4354, -19.385)
  line L10278 (218.0854, -19.985) -> (218.0854, -19.385)
  line L10279 (218.4354, -19.385) -> (218.4354, -19.985)
  line L10280 (214.9854, -77.1606) -> (214.9854, -76.5606)
  line L10281 (214.6354, -76.5606) -> (214.6354, -77.1606)
  line L10282 (214.9854, -76.5606) -> (214.6354, -76.5606)
  line L10283 (214.6354, -77.1606) -> (214.9854, -77.1606)
  line L10284 (218.4354, -77.1606) -> (218.0854, -77.1606)
  line L10285 (218.4354, -76.5606) -> (218.4354, -77.1606)
  line L10286 (218.0854, -77.1606) -> (218.0854, -76.5606)
  line L10287 (218.0854, -76.5606) -> (218.4354, -76.5606)
  line L10288 (214.9854, -57.4978) -> (214.6354, -57.4978)
  line L10289 (214.6354, -57.4978) -> (214.6354, -58.0978)
  line L10290 (214.9854, -58.0978) -> (214.9854, -57.4978)
  line L10291 (214.6354, -58.0978) -> (214.9854, -58.0978)
  line L10292 (218.0854, -57.4978) -> (218.4354, -57.4978)
  line L10293 (218.4354, -58.0978) -> (218.0854, -58.0978)
  line L10294 (218.4354, -57.4978) -> (218.4354, -58.0978)
  line L10295 (218.0854, -58.0978) -> (218.0854, -57.4978)
  line L10296 (214.6354, -39.0351) -> (214.9854, -39.0351)
  line L10297 (214.9854, -39.0351) -> (214.9854, -38.4351)
  line L10298 (214.6354, -38.4351) -> (214.6354, -39.0351)
  line L10299 (214.9854, -38.4351) -> (214.6354, -38.4351)
  line L10300 (218.0854, -39.0351) -> (218.0854, -38.4351)
  line L10301 (218.4354, -39.0351) -> (218.0854, -39.0351)
  line L10302 (218.0854, -38.4351) -> (218.4354, -38.4351)
  line L10303 (218.4354, -38.4351) -> (218.4354, -39.0351)
  line L10304 (195.5854, -38.4351) -> (195.5854, -39.0351)
  line L10305 (195.9354, -39.0351) -> (195.9354, -38.4351)
  line L10306 (195.5854, -39.0351) -> (195.9354, -39.0351)
  line L10307 (195.9354, -38.4351) -> (195.5854, -38.4351)
  line L10308 (199.3854, -39.0351) -> (199.0354, -39.0351)
  line L10309 (199.0354, -39.0351) -> (199.0354, -38.4351)
  line L10310 (199.3854, -38.4351) -> (199.3854, -39.0351)
  line L10311 (199.0354, -38.4351) -> (199.3854, -38.4351)
  line L10312 (195.9354, -77.1606) -> (195.9354, -76.5606)
  line L10313 (195.9354, -76.5606) -> (195.5854, -76.5606)
  line L10314 (195.5854, -77.1606) -> (195.9354, -77.1606)
  line L10315 (195.5854, -76.5606) -> (195.5854, -77.1606)
  line L10316 (199.3854, -77.1606) -> (199.0354, -77.1606)
  line L10317 (199.0354, -76.5606) -> (199.3854, -76.5606)
  line L10318 (199.0354, -77.1606) -> (199.0354, -76.5606)
  line L10319 (199.3854, -76.5606) -> (199.3854, -77.1606)
  line L10320 (195.5854, -57.4978) -> (195.5854, -58.0978)
  line L10321 (195.5854, -58.0978) -> (195.9354, -58.0978)
  line L10322 (195.9354, -57.4978) -> (195.5854, -57.4978)
  line L10323 (195.9354, -58.0978) -> (195.9354, -57.4978)
  line L10324 (199.3854, -57.4978) -> (199.3854, -58.0978)
  line L10325 (199.3854, -58.0978) -> (199.0354, -58.0978)
  line L10326 (199.0354, -58.0978) -> (199.0354, -57.4978)
  line L10327 (199.0354, -57.4978) -> (199.3854, -57.4978)
  line L10328 (195.5854, -19.385) -> (195.5854, -19.985)
  line L10329 (195.9354, -19.985) -> (195.9354, -19.385)
  line L10330 (195.5854, -19.985) -> (195.9354, -19.985)
  line L10331 (195.9354, -19.385) -> (195.5854, -19.385)
  line L10332 (199.3854, -19.985) -> (199.0354, -19.985)
  line L10333 (199.3854, -19.385) -> (199.3854, -19.985)
  line L10334 (199.0354, -19.385) -> (199.3854, -19.385)
  line L10335 (199.0354, -19.985) -> (199.0354, -19.385)
  line L10336 (203.2384, -4.21) -> (202.9384, -4.21)
  line L10337 (202.9384, -3.41) -> (203.2384, -3.41)
  line L10338 (202.9384, -4.21) -> (202.9384, -3.41)
  line L10339 (203.2384, -3.41) -> (203.2384, -4.21)
  line L10340 (201.6384, -4.21) -> (201.9384, -4.21)
  line L10341 (201.9384, -3.41) -> (201.6384, -3.41)
  line L10342 (201.9384, -4.21) -> (201.9384, -3.41)
  line L10343 (201.6384, -3.41) -> (201.6384, -4.21)
  line L10344 (201.0334, -7.131) -> (201.0334, -6.331)
  line L10345 (201.0334, -6.331) -> (201.3334, -6.331)
  line L10346 (201.3334, -6.331) -> (201.3334, -7.131)
  line L10347 (201.3334, -7.131) -> (201.0334, -7.131)
  line L10348 (199.7334, -6.331) -> (199.7334, -7.131)
  line L10349 (200.0334, -7.131) -> (200.0334, -6.331)
  line L10350 (200.0334, -6.331) -> (199.7334, -6.331)
  line L10351 (199.7334, -7.131) -> (200.0334, -7.131)
  line L10352 (205.2404, -5.226) -> (204.9404, -5.226)
  line L10353 (204.9404, -5.226) -> (204.9404, -4.426)
  line L10354 (205.2404, -4.426) -> (205.2404, -5.226)
  line L10355 (204.9404, -4.426) -> (205.2404, -4.426)
  line L10356 (206.2404, -5.226) -> (206.5404, -5.226)
  line L10357 (206.5404, -5.226) -> (206.5404, -4.426)
  line L10358 (206.2404, -4.426) -> (206.2404, -5.226)
  line L10359 (206.5404, -4.426) -> (206.2404, -4.426)
  arc A2468 (10.2131, -8.0011) -> (9.1131, -8.0011) centre (9.6631, -8.0011) ccw
  arc A2469 (9.1131, -8.0011) -> (10.2131, -8.0011) centre (9.6631, -8.0011) ccw
  arc A2470 (10.2131, -5.4611) -> (9.1131, -5.4611) centre (9.6631, -5.4611) ccw
  arc A2471 (9.1131, -5.4611) -> (10.2131, -5.4611) centre (9.6631, -5.4611) ccw
  arc A2472 (10.2131, -2.9211) -> (9.1131, -2.9211) centre (9.6631, -2.9211) ccw
  arc A2473 (9.1131, -2.9211) -> (10.2131, -2.9211) centre (9.6631, -2.9211) ccw
  arc A2474 (-5.3871, -8.0011) -> (-4.287, -8.0011) centre (-4.8371, -8.0011) ccw
  arc A2475 (-4.287, -8.0011) -> (-5.3871, -8.0011) centre (-4.8371, -8.0011) ccw
  arc A2476 (-5.3871, -2.9211) -> (-4.287, -2.9211) centre (-4.8371, -2.9211) ccw
  arc A2477 (-4.287, -2.9211) -> (-5.3871, -2.9211) centre (-4.8371, -2.9211) ccw
  line L10360 (2.9129, -0.5611) -> (1.413, -0.5611)
  line L10361 (2.9129, 0.6389) -> (2.9129, -0.5611)
  line L10362 (1.413, -0.5611) -> (1.413, 0.6389)
  line L10363 (1.413, 0.6389) -> (2.9129, 0.6389)
  line L10364 (2.9129, -11.5611) -> (1.413, -11.5611)
  line L10365 (2.9129, -10.3611) -> (2.9129, -11.5611)
  line L10366 (1.413, -10.3611) -> (2.9129, -10.3611)
  line L10367 (1.413, -11.5611) -> (1.413, -10.3611)
  line L10368 (197.1222, -3.67) -> (197.4822, -3.67)
  line L10369 (197.4822, -3.67) -> (197.4822, -3.92)
  line L10370 (197.1222, -3.92) -> (197.1222, -3.67)
  line L10371 (197.4822, -3.92) -> (197.1222, -3.92)
  line L10372 (197.1223, -5.22) -> (197.1223, -4.97)
  line L10373 (197.4823, -5.22) -> (197.1223, -5.22)
  line L10374 (197.1223, -4.97) -> (197.4823, -4.97)
  line L10375 (197.4823, -4.97) -> (197.4823, -5.22)
  line L10376 (195.5524, -3.67) -> (195.5524, -3.92)
  line L10377 (195.1924, -3.92) -> (195.1924, -3.67)
  line L10378 (195.5524, -3.92) -> (195.1924, -3.92)
  line L10379 (195.1924, -3.67) -> (195.5524, -3.67)
  line L10380 (195.5524, -4.32) -> (195.5524, -4.57)
  line L10381 (195.1924, -4.57) -> (195.1924, -4.32)
  line L10382 (195.1924, -4.32) -> (195.5524, -4.32)
  line L10383 (195.5524, -4.57) -> (195.1924, -4.57)
  line L10384 (195.5524, -5.22) -> (195.1924, -5.22)
  line L10385 (195.1924, -5.22) -> (195.1924, -4.97)
  line L10386 (195.5524, -4.97) -> (195.5524, -5.22)
  line L10387 (195.1924, -4.97) -> (195.5524, -4.97)
  arc A2478 (176.5223, -4.318) -> (175.5224, -4.318) centre (176.0224, -4.318) ccw
  arc A2479 (175.5224, -4.318) -> (176.5223, -4.318) centre (176.0224, -4.318) ccw
  arc A2480 (173.9823, -4.318) -> (172.9824, -4.318) centre (173.4823, -4.318) ccw
  arc A2481 (172.9824, -4.318) -> (173.9823, -4.318) centre (173.4823, -4.318) ccw
  line L10388 (201.4604, -2.305) -> (199.8604, -2.305)
  line L10389 (199.8604, -2.305) -> (199.8604, -1.505)
  line L10390 (199.8604, -1.505) -> (201.4604, -1.505)
  line L10391 (201.4604, -1.505) -> (201.4604, -2.305)
  line L10392 (207.5745, -12.2629) -> (207.5745, -5.2629)
  line L10393 (207.5745, -5.2629) -> (214.5745, -5.2629)
  line L10394 (214.5745, -5.2629) -> (214.5745, -12.2629)
  line L10395 (214.5745, -12.2629) -> (207.5745, -12.2629)
  line L10396 (186.9064, -6.331) -> (188.5064, -6.331)
  line L10397 (186.9064, -7.131) -> (186.9064, -6.331)
  line L10398 (188.5064, -6.331) -> (188.5064, -7.131)
  line L10399 (188.5064, -7.131) -> (186.9064, -7.131)
  line L10400 (183.9344, -7.131) -> (182.3344, -7.131)
  line L10401 (183.9344, -6.331) -> (183.9344, -7.131)
  line L10402 (182.3344, -6.331) -> (183.9344, -6.331)
  line L10403 (182.3344, -7.131) -> (182.3344, -6.331)
  line L10404 (211.6854, -3.786) -> (208.6854, -3.786)
  line L10405 (208.6854, -0.786) -> (211.6854, -0.786)
  line L10406 (211.6854, -0.786) -> (211.6854, -3.786)
  line L10407 (208.6854, -3.786) -> (208.6854, -0.786)
  line L10408 (138.9853, -77.7106) -> (141.6853, -77.7106)
  line L10409 (138.9853, -76.0106) -> (138.9853, -77.7106)
  line L10410 (141.6853, -76.0106) -> (138.9853, -76.0106)
  line L10411 (141.6853, -77.7106) -> (141.6853, -76.0106)
  line L10412 (138.9853, -20.535) -> (141.6853, -20.535)
  line L10413 (138.9853, -18.835) -> (138.9853, -20.535)
  line L10414 (141.6853, -20.535) -> (141.6853, -18.835)
  line L10415 (141.6853, -18.835) -> (138.9853, -18.835)
  line L10416 (138.9853, -37.8851) -> (138.9853, -39.5851)
  line L10417 (138.9853, -39.5851) -> (141.6853, -39.5851)
  line L10418 (141.6853, -37.8851) -> (138.9853, -37.8851)
  line L10419 (141.6853, -39.5851) -> (141.6853, -37.8851)
  line L10420 (141.6853, -56.9478) -> (138.9853, -56.9478)
  line L10421 (138.9853, -56.9478) -> (138.9853, -58.6478)
  line L10422 (141.6853, -58.6478) -> (141.6853, -56.9478)
  line L10423 (138.9853, -58.6478) -> (141.6853, -58.6478)
  line L10424 (158.0353, -20.535) -> (160.7353, -20.535)
  line L10425 (160.7353, -20.535) -> (160.7353, -18.835)
  line L10426 (160.7353, -18.835) -> (158.0353, -18.835)
  line L10427 (158.0353, -18.835) -> (158.0353, -20.535)
  line L10428 (158.0353, -76.0106) -> (158.0353, -77.7106)
  line L10429 (160.7353, -76.0106) -> (158.0353, -76.0106)
  line L10430 (158.0353, -77.7106) -> (160.7353, -77.7106)
  line L10431 (160.7353, -77.7106) -> (160.7353, -76.0106)
  line L10432 (158.0353, -58.6478) -> (160.7353, -58.6478)
  line L10433 (160.7353, -56.9478) -> (158.0353, -56.9478)
  line L10434 (158.0353, -56.9478) -> (158.0353, -58.6478)
  line L10435 (160.7353, -58.6478) -> (160.7353, -56.9478)
  line L10436 (160.7353, -37.8851) -> (158.0353, -37.8851)
  line L10437 (158.0353, -39.5851) -> (160.7353, -39.5851)
  line L10438 (158.0353, -37.8851) -> (158.0353, -39.5851)
  line L10439 (160.7353, -39.5851) -> (160.7353, -37.8851)
  line L10440 (179.7854, -20.535) -> (179.7854, -18.835)
  line L10441 (179.7854, -18.835) -> (177.0854, -18.835)
  line L10442 (177.0854, -20.535) -> (179.7854, -20.535)
  line L10443 (177.0854, -18.835) -> (177.0854, -20.535)
  line L10444 (179.7854, -77.7106) -> (179.7854, -76.0106)
  line L10445 (177.0854, -76.0106) -> (177.0854, -77.7106)
  line L10446 (179.7854, -76.0106) -> (177.0854, -76.0106)
  line L10447 (177.0854, -77.7106) -> (179.7854, -77.7106)
  line L10448 (177.0854, -56.9478) -> (177.0854, -58.6478)
  line L10449 (179.7854, -56.9478) -> (177.0854, -56.9478)
  line L10450 (177.0854, -58.6478) -> (179.7854, -58.6478)
  line L10451 (179.7854, -58.6478) -> (179.7854, -56.9478)
  line L10452 (179.7854, -39.5851) -> (179.7854, -37.8851)